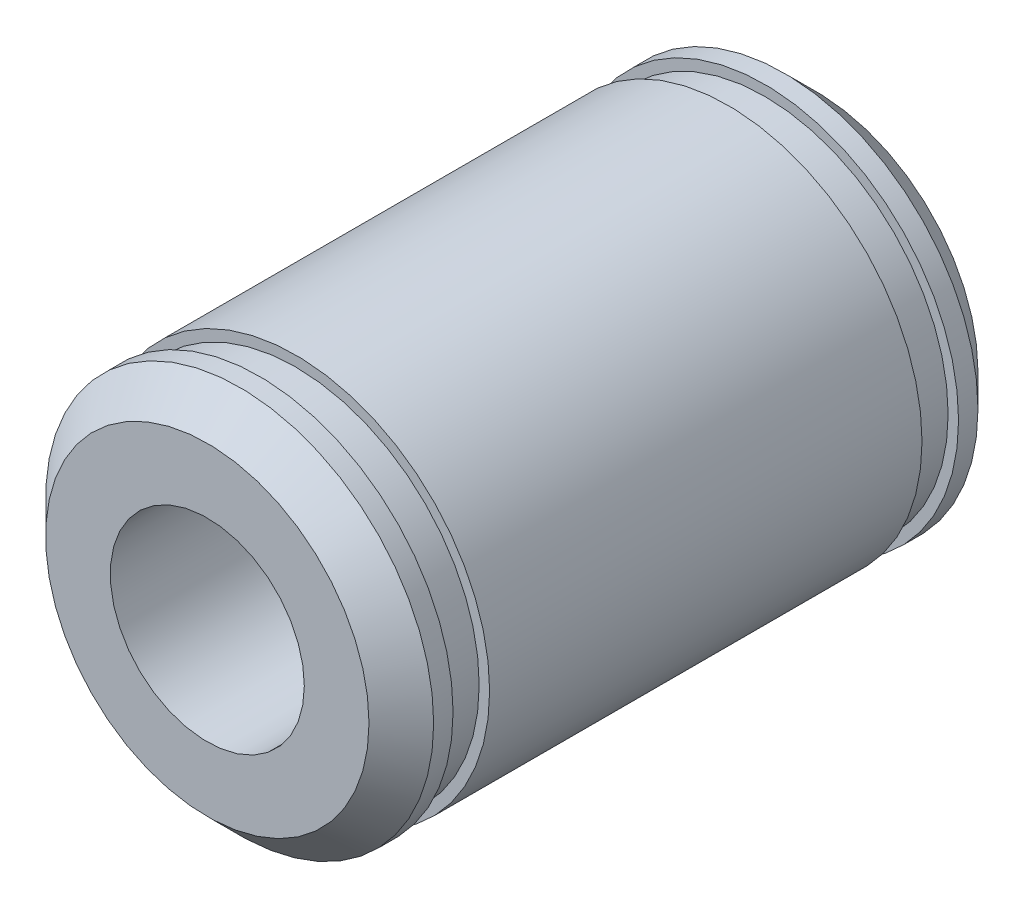
# Autodesk Inventor part: 00_Igus_Drylin_6mm
Saved by Autodesk Inventor 2019.4 (Build 234330000, 330)
## iProperties
Created: 2021-05-03
Part Number: 00_Igus_Drylin_6mm
Material: Generic
Document SubType Name: Modeling
Designer: diederichbenedict
Density: 1 g/cm^3
Appearance: Default
Author: diederichbenedict
Autodesk Inventor part; units mm, degrees
ref_plane "YZ Plane" through (0, 0, 0) normal (1, 0, 0) x (0, 1, 0)
ref_plane "XZ Plane" through (0, 0, 0) normal (0, 1, 0) x (-1, 0, 0)
ref_plane "XY Plane" through (0, 0, 0) normal (0, 0, 1) x (1, 0, 0)
sketch "Sketch1" plane through (0, 0, 0) normal (0, 0, 1) x (1, 0, 0)
  circle A0 centre (0, 0) radius 3
  circle A1 centre (0, 0) radius 6
  dimension "d0" = 6
  dimension "d1" = 12
  constraints: 2 centre point, 2 coincident
  measures "d0" diameter of A0
  measures "d1" diameter of A1
extrude "Extrusion1" add sketch "Sketch1" along normal blind 18.83
chamfer "Chamfer1" distance 1 angle 45 2 edges at (-6, 0, 18.83) (-6, 0, 0)
sketch "Sketch2" plane through (0, 0, 0) normal (1, 0, 0) x (0, 1, 0)
  line L0 (6.8077, 17.23) -> (5.6777, 17.23)
  line L1 (5.6777, 17.23) -> (5.6777, 16.1)
  line L2 (5.6777, 16.1) -> (6.8077, 16.1)
  line L3 (6.8077, 16.1) -> (6.8077, 17.23)
  line L4 (-5, 18.83) -> (5, 18.83) projected
  line L5 (6.8077, 1.6) -> (5.6777, 1.6)
  line L6 (5.6777, 1.6) -> (5.6777, 2.73)
  line L7 (5.6777, 2.73) -> (6.8077, 2.73)
  line L8 (6.8077, 2.73) -> (6.8077, 1.6)
  line L9 (5, 0) -> (-5, 0) projected
  line L10 (0, -3.766) -> (0, 22.596) projected
  point P0 (0, 0)
  dimension "d7" = 1.13
  dimension "d8" = 1.13
  dimension "d9" = 1.6
  dimension "d10" = 1.13
  dimension "d11" = 1.13
  dimension "d12" = 1.6
  constraints: 16 end point, 4 parallel, 2 horizontal, 2 perpendicular
  measures "d7" distance of L2.end L1.end
  measures "d8" distance of L1.end L0.end
  measures "d9" distance between parallel lines of L0 L4
  measures "d10" distance of L6.end L7.end
  measures "d11" distance of L5.end L6.end
  measures "d12" distance between parallel lines of L5 L9
revolve "Revolution1" cut sketch "Sketch2" angle 360 about axis through (0, 0, -10) along (0, 0, 1)
body "Solid1"
